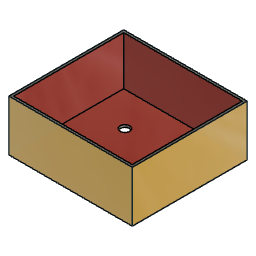
Box_for_inductor v2 (Autodesk Fusion 360 design; units mm, degrees)
Autodesk Fusion 360 part; units mm, degrees
box "BoxPrimitive1" add length 47.33 width 50.88 height 21 placed x (0, 1, 0) y (-1, 0, 0) z (0, 0, 1) at (50.88, 0, 0)
shell "Shell1" thickness 1 removed faces 1 at (16.96, 15.7767, 21)
sketch "Sketch2" plane through (0, 0, 0) normal (0, 0, 1) x (1, 0, 0)
  circle A0 centre (35.5, 11.5) radius 2
  circle A1 centre (15.5, 11.5) radius 2
  circle A2 centre (35.5, 32.3244) radius 2
  circle A3 centre (15.5, 32.3244) radius 2
  dimension "d11" = 4
  dimension "d12" = 4
  dimension "d15" = 4
  dimension "d16" = 4
  measures "d11" diameter of A0
  measures "d12" diameter of A1
  measures "d15" diameter of A2
  measures "d16" diameter of A3
extrude "Extrude1" cut sketch "Sketch2" along normal blind 15
sketch "Sketch3" plane through (0, 0, 0) normal (-1, 0, 0) x (0, -1, 0)
  line L0 (-47.33, 21) -> (-47.33, 0)
  line L1 (-47.33, 0) -> (0, 0)
  line L2 (0, 0) -> (0, 21)
  line L3 (0, 21) -> (-47.33, 21)
  line L4 (-26.8184, 16.7615) -> (-19.8184, 16.7615)
  line L5 (-19.8184, 16.7615) -> (-19.8184, 12.7615)
  line L6 (-19.8184, 12.7615) -> (-26.8184, 12.7615)
  line L7 (-26.8184, 12.7615) -> (-26.8184, 16.7615)
  line L8 (-26.8184, 6.7615) -> (-19.8184, 6.7615)
  line L9 (-19.8184, 2.7615) -> (-26.8184, 2.7615)
  line L10 (-26.8184, 2.7615) -> (-26.8184, 6.7615)
  line L11 (-19.8184, 6.7615) -> (-19.8184, 2.7615)
  line L12 (-26.8184, 2.7615) -> (-26.8184, 6.7615)
  line L13 (-26.8184, 16.7615) -> (-19.8184, 16.7615)
  line L14 (-19.8184, 16.7615) -> (-19.8184, 12.7615)
  line L15 (-26.8184, 6.7615) -> (-19.8184, 6.7615)
  line L16 (-19.8184, 12.7615) -> (-26.8184, 12.7615)
  line L17 (-26.8184, 12.7615) -> (-26.8184, 16.7615)
  line L18 (-19.8184, 6.7615) -> (-19.8184, 2.7615)
  line L19 (-19.8184, 2.7615) -> (-26.8184, 2.7615)
  constraint horizontal L4
  constraint vertical L5
  constraint horizontal L6
  constraint vertical L7
  constraint horizontal L8
  constraint vertical L11
  constraint horizontal L9
  constraint vertical L10
  constraint horizontal L13
  constraint vertical L14
  constraint horizontal L16
  constraint vertical L17
  constraint horizontal L15
  constraint vertical L18
  constraint horizontal L19
  constraint vertical L12
extrude "Extrude2" cut sketch "Sketch3" against normal blind 100 contours L4 L5 L6 L7 L13 L14 L16 L17 | L8 L9 L10 L11 L12 L15 L18 L19
sketch "Sketch4" plane through (0, 47.33, 0) normal (0, 1, 0) x (-1, 0, 0)
  line L0 (-50.88, 21) -> (-50.88, 0)
  line L1 (-50.88, 0) -> (0, 0)
  line L2 (0, 0) -> (0, 21)
  line L3 (0, 21) -> (-50.88, 21)
  line L4 (-30, 17) -> (-23, 17)
  line L5 (-23, 17) -> (-23, 13)
  line L6 (-23, 13) -> (-30, 13)
  line L7 (-30, 13) -> (-30, 17)
  line L8 (-30, 6.76) -> (-23, 6.76)
  line L9 (-30, 2.76) -> (-30, 6.76)
  line L10 (-23, 6.76) -> (-23, 2.76)
  line L11 (-23, 2.76) -> (-30, 2.76)
  dimension "d24" = 2.76
  constraint horizontal L4
  constraint vertical L5
  constraint horizontal L6
  constraint vertical L7
  constraint horizontal L8
  constraint vertical L10
  constraint horizontal L11
  constraint vertical L9
  measures "d24" distance of L1 L10.end
sketch "Sketch5" plane through (50.88, 0, 0) normal (1, 0, 0) x (0, 1, 0)
  line L0 (0, 21) -> (0, 0)
  line L1 (0, 0) -> (47.33, 0)
  line L2 (47.33, 0) -> (47.33, 21)
  line L3 (47.33, 21) -> (0, 21)
extrude "Extrude3" cut sketch "Sketch4" against normal blind 100 contours L4 L5 L6 L7 | L8 L9 L10 L11
sketch "Sketch6" plane through (0, 0, 0) normal (0, -1, 0) x (1, 0, 0)
  line L0 (0, 21) -> (0, 0)
  line L1 (0, 0) -> (50.88, 0)
  line L2 (50.88, 0) -> (50.88, 21)
  line L3 (50.88, 21) -> (0, 21)
sketch "Sketch7" plane through (0, 0, 0) normal (0, 1, 0) x (1, 0, 0)
  line L0 (21.5384, -18.6538) -> (31.923, -18.6538)
  line L1 (31.923, -18.6538) -> (31.923, -1.2179)
  line L2 (31.923, -1.2179) -> (21.5384, -1.2179)
  line L3 (21.5384, -1.2179) -> (21.5384, -18.6538)
  constraint horizontal L0
  constraint vertical L1
  constraint horizontal L2
  constraint vertical L3
extrude "Extrude4" add sketch "Sketch7" along normal blind 1
sketch "Sketch8" plane through (50.88, 0, 0) normal (1, 0, 0) x (0, 1, 0)
  line L0 (16.4102, 19.1666) -> (31.4102, 19.1666)
  line L1 (31.4102, 19.1666) -> (31.4102, 1.2179)
  line L2 (31.4102, 1.2179) -> (16.4102, 1.2179)
  line L3 (16.4102, 1.2179) -> (16.4102, 19.1666)
  constraint horizontal L0
  constraint vertical L1
  constraint horizontal L2
  constraint vertical L3
extrude "Extrude5" add sketch "Sketch8" against normal blind 1
sketch "Sketch9" plane through (0, 47.33, 0) normal (0, 1, 0) x (-1, 0, 0)
  line L0 (-50.88, 21) -> (-50.88, 0)
  line L1 (-50.88, 0) -> (0, 0)
  line L2 (0, 0) -> (0, 21)
  line L3 (0, 21) -> (-50.88, 21)
delete_face "DeleteFace1" 8 faces at (27.6667, 46.9967, 17) (25.3333, 46.9967, 13) (25.3333, 46.9967, 2.76) (27.6667, 46.9967, 6.76) (23, 46.9967, 5.4267) (30, 46.9967, 14.3333) (23, 46.9967, 15.6667) (30, 46.9967, 4.0933)
sketch "Sketch10" plane through (0, 0, 0) normal (-1, 0, 0) x (0, -1, 0)
  line L0 (-47.33, 21) -> (-47.33, 0)
  line L1 (-47.33, 0) -> (0, 0)
  line L2 (0, 0) -> (0, 21)
  line L3 (0, 21) -> (-47.33, 21)
delete_face "DeleteFace2" 8 faces at (0.3333, 24.4851, 6.7615) (0.3333, 26.8184, 14.0948) (0.3333, 19.8184, 5.4282) (0.3333, 22.1517, 2.7615) (0.3333, 24.4851, 16.7615) (0.3333, 26.8184, 4.0948) (0.3333, 22.1517, 12.7615) (0.3333, 19.8184, 15.4282)
